# Autodesk Inventor part: Part2
Saved by Autodesk Inventor 2016 (Build 200138000, 138)
## iProperties
Created: 2016-09-04
Part Number: Part2
Material: Steel, Carbon
Document SubType Name: Modeling
Designer: gus
Density: 7.85 g/cm^3
Appearance: Semi-Polished
Author: gus
Autodesk Inventor part; units mm, degrees
ref_plane "YZ Plane" through (0, 0, 0) normal (1, 0, 0) x (0, 1, 0)
ref_plane "XZ Plane" through (0, 0, 0) normal (0, 1, 0) x (-1, 0, 0)
ref_plane "XY Plane" through (0, 0, 0) normal (0, 0, 1) x (1, 0, 0)
sketch "Sketch1" plane through (0, 0, 0) normal (1, 0, 0) x (0, 1, 0)
  circle A0 centre (0, 0) radius 6.35
  dimension "d0" = 12.7
  constraints: 1 centre point, 1 coincident
  measures "d0" diameter of A0
extrude "Extrusion1" add sketch "Sketch1" along normal blind 228.6
sketch "Sketch2" plane through (228.6, 0, 0) normal (1, 0, 0) x (0, 0, -1)
  line L0 (-6.35, 9.525) -> (6.35, 9.525)
  line L1 (6.35, 9.525) -> (6.35, -9.525)
  line L2 (6.35, -9.525) -> (-6.35, -9.525)
  line L3 (-6.35, -9.525) -> (-6.35, 9.525)
  point P0 (0, 0)
  dimension "d3" = 19.05
  dimension "d4" = 12.7
  dimension "d5" = 9.525
  dimension "d6" = 6.35
  constraints: 8 end point, 2 parallel, 1 horizontal, 1 perpendicular
  measures "d3" distance between parallel lines of L0 L2
  measures "d4" distance of L0.start L0.end
  measures "d5" distance from line of point (0, 0) L0
  measures "d6" distance from line of point (0, 0) L1
extrude "Extrusion2" add sketch "Sketch2" along normal blind 38.1
sketch "Sketch3" plane through (228.6, -9.525, 6.35) normal (0, 0, 1) x (1, 0, 0)
  circle A0 centre (25.4, 9.525) radius 6.35
  line L0 (0, 19.05) -> (38.1, 19.05) projected
  line L1 (38.1, 19.05) -> (38.1, 0) projected
  point P0 (-228.6, 9.525)
  dimension "d9" = 12.7
  dimension "d10" = 9.525
  dimension "d11" = 12.7
  constraints: 1 centre point
  measures "d9" diameter of A0
  measures "d10" distance from line of L0 A0.centre
  measures "d11" distance from line of L1 A0.centre
extrude "Extrusion3" cut sketch "Sketch3" against normal blind 38.1
fillet "Fillet1" radius 3.175 13 edges at (247.65, 9.525, 6.35) (247.65, 9.525, -6.35) (228.6, -4.7625, 6.35) (228.6, 4.7625, 6.35) (228.6, 9.525, 0) (247.65, -9.525, 6.35) (266.7, -9.525, 0) (266.7, 0, 6.35) (266.7, 0, -6.35) (247.65, -9.525, -6.35) (228.6, -4.7625, -6.35) (228.6, 4.7625, -6.35) (266.7, 9.525, 0)
body "Solid1"
